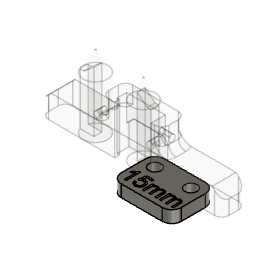
Pittsburgh Caliper Accessories (Autodesk Fusion 360 design; units mm, degrees)
Autodesk Fusion 360 part; units mm, degrees
cylinder "CylinderPrimitive1" add diameter 10 height 30 placed x (1, 0, 0) y (0, 1, 0) z (0, 0, 1) at (0, 0, 0) makes body 1 in component "Pins (Print 2)"
sketch "Sketch C2C Pin Slot" plane through (0, 0, 0) normal (0, 0, -1) x (1, 0, 0) in component "Pins (Print 2)"
  circle A0 centre (0, 0) radius 5
  line L0 (0, 0) -> (5, 0) construction
  line L1 (0, 1.65) -> (4.7199, 1.65)
  line L2 (0, -1.65) -> (4.7199, -1.65)
  line L3 (0, 1.65) -> (0, -1.65)
  line L4 (0, -1.65) -> (-1, -1.65)
  line L5 (-1, -1.65) -> (-1, 1.65)
  line L6 (0, 1.65) -> (-1, 1.65)
  dimension "d3" = 3.3
  dimension "d72" = 6
  constraint coincident A0.centre L0.start
  constraint coincident A0 L0.end
  constraint horizontal L0
  constraint coincident A0 L1.end
  constraint symmetric L0 L1.start L2.start
  constraint symmetric L0 L1.end L2.end
  constraint perpendicular L3 L4
  constraint perpendicular L1 L5
  constraint perpendicular L5 L6
  constraint collinear L2 L4
  measures "d3" distance of L1 L2
  measures "d72" horizontal distance of L0.end L4.end
extrude "Extrude1" cut sketch "Sketch C2C Pin Slot" against normal blind 25 contours A0 L1 L2 L3 | L3 L4 L5 L6 bodies 1 in component "Pins (Print 2)"
draft "Draft1" angle -40 neutral plane through (-1, 1.65, 0) pull (1, 0, 0) 1 faces at (1, 0, 25) on bodies 1 in component "Pins (Print 2)"
chamfer "Chamfer1" distance 4.7 angle 60 1 edges at (-4.6616, -1.8081, 30) measured on face at (1.3101, -1.9935, 30) on bodies 1 in component "Pins (Print 2)"
ref_plane "WorkPlane1" through (0, 5, 15.0265) normal (0, 1, 0) x (1, 0, 0) in component "Pins (Print 2)"
sketch "Sketch C2C Screw Hole" plane through (0, 5, 0) normal (0, 1, 0) x (1, 0, 0) in component "Pins (Print 2)"
  line L0 (0.3, -30) -> (-0.3, -30)
  line L1 (4.7199, 0) -> (-5, 0)
  line L2 (4.7199, 0) -> (4.7199, -20.2004)
  line L3 (5, -19.9654) -> (4.7199, -20.2004)
  line L4 (0.3, -30) -> (5, -21.8594)
  line L5 (-0.3, -30) -> (-5, -21.8594)
  line L6 (-5, 0) -> (-5, -21.8594)
  line L7 (5, -19.9654) -> (5, -21.8594)
  line L8 (-1, 0) -> (4.7199, 0)
  line L9 (4.7199, 0) -> (4.7199, -20.2004)
  line L10 (4.7199, -20.2004) -> (-1, -25)
  line L11 (1, 0) -> (1, -33.6814) construction
  circle A0 centre (1, -5) radius 1.35
  line L12 (1, -6.9092) -> (0.0454, -5.9546)
  line L13 (1, -6.9092) -> (1.9546, -5.9546)
  line L14 (-1, -25) -> (-1, 0)
  line L15 (-1, -25) -> (-3.1868, -25)
  dimension "d11" = 20
  dimension "d12" = 2.7
  dimension "d73" = 2
  constraint coincident L1 L11.start
  constraint perpendicular L8 L11
  constraint coincident L11 A0.centre
  constraint coincident L11 L12.start
  constraint coincident A0 L12.end
  constraint coincident A0 L13.end
  constraint tangent A0 L13
  constraint tangent A0 L12
  constraint coincident L12.start L13.start
  constraint perpendicular L12 L13
  constraint coincident L10.end L14.start
  constraint coincident L5 L15.end
  constraint perpendicular L14 L15
  measures "d11" vertical distance of L10.end A0.centre
  measures "d12" diameter of A0
  measures "d73" distance of L11 L14
extrude "Extrude2" cut sketch "Sketch C2C Screw Hole" against normal up to surface (3.35 mm away) contours A0 | A0 L12 L13 bodies 1 in component "Pins (Print 2)"
ref_plane "WorkPlane2" through (5, 0, 15.8292) normal (1, 0, 0) x (0, -1, 0) in component "Pins (Print 2)"
sketch "Sketch C2C slot cleanup for 3d printing" plane through (5, 0, 0) normal (1, 0, 0) x (0, 1, 0) in component "Pins (Print 2)"
  line L0 (-1.65, 0) -> (-1.65, 20.2004)
  line L1 (1.65, 20.2004) -> (1.65, 0)
  line L2 (1.65, 20.2004) -> (1.65, 21.513)
  line L3 (1.65, 21.513) -> (-1.65, 21.513)
  line L4 (-1.65, 21.513) -> (-1.65, 20.2004)
  line L5 (1.65, 20.4427) -> (-1.65, 20.4427)
  ellipse E0 centre (0, 24.1609) end of major axis (5, 24.1609) minor radius 4.1955 (-1.65, 20.2004) -> (1.65, 20.2004) ccw
  line L6 (0, 21.8594) -> (0, 19.9654) construction
  line L7 (1.65, 19.9654) -> (-1.65, 19.9654)
  point P0 (0, 21.8594)
  constraint coincident L1.start L2.start
  constraint parallel L1 L2
  constraint perpendicular L0 L3
  constraint coincident L0.end L4.end
  constraint perpendicular L3 L4
  constraint coincident L1 L5.start
  constraint coincident L0 L5.end
  constraint perpendicular L0 L5
  constraint coincident P0 L6.start
  constraint coincident E0 L6.end
  constraint coincident L1 L7.start
  constraint coincident L0 L7.end
  constraint perpendicular L0 L7
  constraint coincident L6.end L7
extrude "Extrude3" cut sketch "Sketch C2C slot cleanup for 3d printing" against normal blind 5 contours L2 L4 L5 E0 | L2 L3 L4 L5 bodies 1 in component "Pins (Print 2)"
mirror "Mirror1" about plane through (0, 0, 0) normal (1, 0, 0) of bodies 1 makes body 2 in component "Pins (Print 2)"
move_body "Move1" bodies 2 to x (1, 0, 0) y (0, 1, 0) z (0, 0, 1) at (-20, 0, 0) in component "Pins (Print 2)"
box "BoxPrimitive1" add length 18 width 25 height 5 placed x (0, -1, 0) y (1, 0, 0) z (0, 0, 1) at (4.716, 0, 0) separate body makes body 3 in component "Calibration Jig"
sketch "Sketch C2C Calibration Jig" plane through (0, 0, 5) normal (0, 0, 1) x (-1, 0, 0) in component "Calibration Jig"
  line L0 (-4.716, 18) -> (-29.716, 18)
  line L1 (-29.716, 18) -> (-29.716, 0)
  line L2 (-29.716, 0) -> (-4.716, 0)
  line L3 (-4.716, 0) -> (-4.716, 18)
  line L4 (-17.216, 18) -> (-17.216, 0) construction
  line L5 (-14.858, 5) -> (-9.716, 5) construction
  circle A0 centre (-9.716, 5) radius 2.5
  circle A1 centre (-24.716, 5) radius 2.5
  line L6 (-4.716, 16) -> (-29.716, 16) construction
  line L7 (-29.716, 16) -> (-29.716, 9.5) construction
  line L8 (-29.716, 9.5) -> (-4.716, 9.5) construction
  line L9 (-4.716, 9.5) -> (-4.716, 16) construction
  line L10 (-9.716, 5) -> (-9.716, 7.5) construction
  point P0 (-28.0837, 11.3799)
  point P1 (-6.3483, 11.3799)
  dimension "d29" = 5
  dimension "d30" = 5
  dimension "d31" = 15
  dimension "d37" = 6
  dimension "d38" = 2
  dimension "d39" = 2
  text T0 "15mm" font "Arial" height 6 align centre middle in box 25 x 6.5 at (-4.716, 16) x (-1, 0) y (0, -1) spacing 1 kerned
  constraint midpoint L0 L4.start
  constraint midpoint L2 L4.end
  constraint perpendicular L4 L5
  constraint coincident L5.end A0.centre
  constraint symmetric L4 A0 A1
  constraint symmetric L4 P0 P1
  constraint coincident L1
  constraint coincident L3
  constraint coincident A0 L10.end
  constraint perpendicular L5 L10
  measures "d29" diameter of A0
  measures "d30" distance of L2 L5
  measures "d31" distance of L5.end A1.centre
  measures "d38" distance of L8 L10.end
  measures "d39" distance of L0 L6
hole "Hole1" at (9.716, -5, 5) at (24.716, -5, 5) direction (0, 0, -1) diameter 5 end up to surface (5 mm away) bodies 3 in component "Calibration Jig"
extrude "Extrude1'" cut sketch "Sketch C2C Calibration Jig" against normal blind 3 text T0 bodies 3 in component "Calibration Jig"
fillet "Fillet1" radius 4 4 edges at (4.716, -18, 2.5) (4.716, 0, 2.5) (29.716, 0, 2.5) (29.716, -18, 2.5) on bodies 3 in component "Calibration Jig"
sketch "Sketch1" plane through (0, 0, 0) normal (0, 1, 0) x (1, 0, 0) in component "Depth Base"
  line L0 (37.5, 0) -> (0, 0)
  line L1 (37.5, 0) -> (37.5, -10)
  line L2 (37.5, -10) -> (12.5, -10)
  line L3 (12.5, -10) -> (12.5, -20)
  line L4 (12.5, -20) -> (0, -20)
  line L5 (0, -20) -> (0, -2.5)
  line L6 (-12.5, -20) -> (0, -20)
  line L7 (-12.5, -10) -> (-12.5, -20)
  line L8 (-37.5, -10) -> (-12.5, -10)
  line L9 (-37.5, 0) -> (0, 0)
  line L10 (-37.5, 0) -> (-37.5, -10)
  dimension "d46" = 10
  dimension "d47" = 20
  dimension "d49" = 25
  dimension "d50" = 75
  constraint coincident L0.end L9.end
  constraint horizontal L0
  constraint perpendicular L0 L1
  constraint perpendicular L1 L2
  constraint perpendicular L2 L3
  constraint perpendicular L3 L4
  constraint symmetric L0.start L5 L9.start
  constraint symmetric L0.end L5 L9.end
  constraint symmetric L1.end L5 L8.start
  constraint symmetric L2.end L5 L7.start
  constraint symmetric L3.end L5 L6.start
  constraint symmetric L4.end L5 L6.end
  measures "d46" distance of L0.start L1.end
  measures "d47" distance of L0 L4
  measures "d49" distance of L3 L6.start
  measures "d50" distance of L0.start L10
extrude "Extrude1''" add sketch "Sketch1" along normal mid plane 10 separate body makes body 4 in component "Depth Base"
sketch "Sketch2" plane through (0, -5, 0) normal (0, -1, 0) x (1, 0, 0) in component "Depth Base"
  line L0 (-37.5, 0) -> (37.5, 0)
  line L1 (37.5, 0) -> (37.5, 10)
  line L2 (37.5, 10) -> (12.5, 10)
  line L3 (12.5, 10) -> (12.5, 20)
  line L4 (12.5, 20) -> (-12.5, 20)
  line L5 (-12.5, 20) -> (-12.5, 10)
  line L6 (-12.5, 10) -> (-37.5, 10)
  line L7 (-37.5, 10) -> (-37.5, 0)
  line L8 (0, 20) -> (0, 0) construction
  line L9 (8.05, 20) -> (8.05, 0)
  line L10 (-8.05, 20) -> (-8.05, 0)
  line L11 (-8.05, 11) -> (8.05, 11)
  line L12 (-7.05, 20) -> (-7.05, 0)
  line L13 (6.05, 11) -> (8.05, 9)
  line L14 (-6.05, 11) -> (-8.05, 9)
  dimension "d53" = 16.1
  dimension "d54" = 11
  dimension "d63" = 1
  dimension "d75" = 45
  dimension "d76" = 2
  constraint midpoint L4 L8.start
  constraint coincident L8.end origin
  constraint coincident L4 L9.start
  constraint coincident L0 L9.end
  constraint perpendicular L0 L9
  constraint symmetric L8 L9.start L10.start
  constraint symmetric L8 L9.end L10.end
  constraint coincident L10 L11.start
  constraint coincident L9 L11.end
  constraint perpendicular L9 L11
  constraint coincident L4 L12.start
  constraint coincident L0 L12.end
  constraint perpendicular L0 L12
  constraint coincident L11 L13.start
  constraint coincident L9 L13.end
  constraint symmetric L8 L13.start L14.start
  constraint symmetric L8 L13.end L14.end
  measures "d53" distance of L9.start L10.start
  measures "d54" distance of L0 L11
  measures "d63" distance of L10 L12
  measures "d75" angle of L11 L13
  measures "d76" distance of L11.end L13.end
extrude "Extrude2'" cut sketch "Sketch2" against normal blind 6 contours L10 L11 L12 L14 | L11 L12 L14 | L4 L10 L11 L12 | L9 L11 L13 | L4 L9 L11 L12 bodies 4 in component "Depth Base"
extrude "Extrude3'" cut sketch "Sketch2" against normal blind 7 contours L0 L10 L12 L14 | L0 L9 L11 L12 L13 L14 bodies 4 in component "Depth Base"
sketch "Sketch3" plane through (12.5, 0, 0) normal (1, 0, 0) x (0, 1, 0) in component "Depth Base"
  line L0 (-5, 10) -> (5, 10)
  line L1 (5, 10) -> (5, 20)
  line L2 (5, 20) -> (-5, 20)
  line L3 (-5, 20) -> (-5, 10)
  line L4 (-5, 20) -> (-5, 0)
  line L5 (-5, 0) -> (2, 0)
  line L6 (2, 0) -> (2, 9)
  line L7 (1, 20) -> (-5, 20)
  circle A0 centre (-0.7, 14.5) radius 1.35
  line L8 (-0.7, 14.5) -> (-0.7, 16.4092) construction
  line L9 (-0.7, 16.4092) -> (0.2546, 15.4546)
  line L10 (-0.7, 16.4092) -> (-1.6546, 15.4546)
  line L11 (0.9, 14.5) -> (-0.7, 14.5) construction
  line L12 (1, 9) -> (1, 20)
  line L13 (2, 9) -> (1, 9)
  dimension "d59" = 2.7
  dimension "d74" = 1.7
  constraint coincident A0.centre L8.start
  constraint vertical L8
  constraint coincident A0 L9.end
  constraint tangent A0 L9
  constraint symmetric L9.start L8 L10.start
  constraint symmetric L8 L9.end L10.end
  constraint perpendicular L9 L10
  constraint horizontal L11
  measures "d59" diameter of A0
  measures "d74" distance of A0.centre L12
extrude "Extrude4" cut sketch "Sketch3" against normal blind 4.45 contours A0 | A0 L9 L10 bodies 4 in component "Depth Base"
extrude "Extrude5" add sketch "Sketch2" against normal blind 2 contours L0 L10 L12 L14 | L10 L11 L12 L14 | L4 L10 L11 L12 bodies 4 in component "Depth Base"
chamfer "Chamfer1'" distance 1 angle 45 1 edges at (0, 1, 11) on bodies 4 in component "Depth Base"
chamfer "Chamfer2" distance 4 angle 45 2 edges at (-37.5, 0, 10) (37.5, 0, 10) on bodies 4 in component "Depth Base"
fillet "Fillet1'" radius 3 8 edges at (-37.5, -5, 3) (37.5, -5, 3) (37.5, 5, 3) (-37.5, 5, 3) (-12.5, 5, 15) (12.5, 5, 15) (-12.5, -5, 15) (12.5, -5, 15) on bodies 4 in component "Depth Base"
fillet "Fillet2" radius 3 6 edges at (-11.6213, -4.1213, 10) (-12.5, 0, 10) (-11.6213, 4.1213, 10) (11.6213, -4.1213, 10) (12.5, 0, 10) (11.6213, 4.1213, 10) on bodies 4 in component "Depth Base"
move_body "Move1'" [rolled back] in component "Depth Base"
component "Depth Base" placed x (1, 0, 0) y (0, 1, 0) z (0, 0, 1) at (0, 0, 0)
component "Radius Base" placed x (1, 0, 0) y (0, 1, 0) z (0, 0, 1) at (0, 0, 0)
component "Center to Center Measuring" placed x (1, 0, 0) y (0, 1, 0) z (0, 0, 1) at (0, 0, 0)
component "Calibration Jig" placed x (1, 0, 0) y (0, 1, 0) z (0, 0, 1) at (0, 0, 0) in component "Center to Center Measuring"
component "Pins (Print 2)" placed x (1, 0, 0) y (0, 1, 0) z (0, 0, 1) at (0, 0, 0) in component "Center to Center Measuring"
equation "d50 = DepthBaseLength"
equation "DepthBaseLength = 75 mm"
named bodies: "C2C Pin - Original", "C2C Pin - Mirror", "C2C  Calibration Jig", "Depth Measuring Base"
